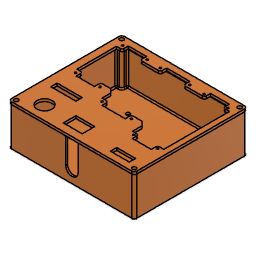
PCB Box v1 (Autodesk Fusion 360 design; units mm, degrees)
Autodesk Fusion 360 part; units mm, degrees
sketch "Sketch1" plane through (0, 0, 0) normal (0, 1, 0) x (1, 0, 0) in component "PCB_Faceplate"
  line L0 (-50, 45) -> (50, 45)
  line L1 (50, 45) -> (50, -45)
  line L2 (50, -45) -> (-50, -45)
  line L3 (-50, -45) -> (-50, 45)
  line L4 (-42.25, 38) -> (-22.75, 38) construction
  line L5 (-22.75, 38) -> (-22.75, 0.5) construction
  line L6 (-22.75, 0.5) -> (-42.25, 0.5) construction
  line L7 (-42.25, 0.5) -> (-42.25, 38) construction
  line L8 (-11.75, 37.5) -> (11.75, 37.5) construction
  line L9 (11.75, 37.5) -> (11.75, -9) construction
  line L10 (11.75, -9) -> (-11.75, -9) construction
  line L11 (-11.75, -9) -> (-11.75, 37.5) construction
  line L12 (23.75, 36.875) -> (42.75, 36.875) construction
  line L13 (42.75, 36.875) -> (42.75, -19.125) construction
  line L14 (42.75, -19.125) -> (23.75, -19.125) construction
  line L15 (23.75, -19.125) -> (23.75, 36.875) construction
  line L16 (-50, -45) -> (50, 45) construction
  circle A0 centre (-42.25, 38) radius 0.8
  circle A1 centre (-22.75, 38) radius 0.8
  circle A2 centre (-42.25, 0.5) radius 0.8
  circle A3 centre (-22.75, 0.5) radius 0.8
  circle A4 centre (-11.75, -9) radius 0.8
  circle A5 centre (11.75, -9) radius 0.8
  circle A6 centre (11.75, 37.5) radius 0.8
  circle A7 centre (-11.75, 37.5) radius 0.8
  circle A8 centre (23.75, 36.875) radius 0.8
  circle A9 centre (42.75, 36.875) radius 0.8
  circle A10 centre (42.75, -19.125) radius 0.8
  circle A11 centre (23.75, -19.125) radius 0.8
  line L17 (-44.25, 40) -> (-20.75, 40)
  line L18 (-20.75, 40) -> (-20.75, -1.5)
  line L19 (-20.75, -1.5) -> (-44.25, -1.5)
  line L20 (-44.25, -1.5) -> (-44.25, 40)
  line L21 (-14.25, 40) -> (14.25, 40)
  line L22 (14.25, 40) -> (14.25, -11.5)
  line L23 (14.25, -11.5) -> (-14.25, -11.5)
  line L24 (-14.25, -11.5) -> (-14.25, 40)
  line L25 (20.75, 40) -> (45.75, 40)
  line L26 (45.75, 40) -> (45.75, -22.25)
  line L27 (45.75, -22.25) -> (20.75, -22.25)
  line L28 (20.75, -22.25) -> (20.75, 40)
  line L29 (20.75, -22.25) -> (45.75, 40) construction
  line L30 (-14.25, -11.5) -> (14.25, 40) construction
  line L31 (-44.25, -1.5) -> (-20.75, 40) construction
  line L32 (-22.75, 0.5) -> (-42.25, 38) construction
  line L33 (-11.75, 37.5) -> (11.75, -9) construction
  line L34 (23.75, 36.875) -> (42.75, -19.125) construction
  line L35 (-20.75, 40) -> (-14.25, 40)
  line L36 (14.25, 40) -> (20.75, 40)
  line L37 (0, -45) -> (0, 45) construction
  line L38 (0, 14.25) -> (11.75, 14.25) construction
  line L39 (9.25, -11.5) -> (9.25, -6.5)
  line L40 (9.25, -6.5) -> (14.25, -6.5)
  line L41 (-9.25, -11.5) -> (-9.25, -6.5)
  line L42 (-9.25, -6.5) -> (-14.25, -6.5)
  line L43 (-25.25, -1.5) -> (-25.25, 3.5)
  line L44 (-25.25, 3.5) -> (-20.75, 3.5)
  line L45 (-39.75, -1.5) -> (-39.75, 3.5)
  line L46 (-39.75, 3.5) -> (-44.25, 3.5)
  line L47 (-44.25, 35) -> (-39.75, 35)
  line L48 (-39.75, 35) -> (-39.75, 40)
  line L49 (-25.25, 40) -> (-25.25, 35)
  line L50 (-25.25, 35) -> (-20.75, 35)
  line L51 (-14.25, 35) -> (-9.25, 35)
  line L52 (-9.25, 35) -> (-9.25, 40)
  line L53 (9.25, 40) -> (9.25, 35)
  line L54 (9.25, 35) -> (14.25, 35)
  line L55 (20.75, 35) -> (25.75, 35)
  line L56 (25.75, 35) -> (25.75, 40)
  line L57 (40.75, 40) -> (40.75, 35)
  line L58 (40.75, 35) -> (45.75, 35)
  line L59 (40.75, -22.25) -> (40.75, -17.25)
  line L60 (40.75, -17.25) -> (45.75, -17.25)
  line L61 (20.75, -17.25) -> (25.75, -17.25)
  line L62 (25.75, -17.25) -> (25.75, -22.25)
  line L63 (-20.75, 3.5) -> (-14.25, 3.5)
  line L64 (14.25, -6.5) -> (20.75, -6.5)
  line L65 (-14.25, 35) -> (-20.75, 35)
  line L66 (20.75, 35) -> (14.25, 35)
  line L67 (-42.5, -14) -> (-22.5, -14)
  line L68 (-22.5, -14) -> (-22.5, -19)
  line L69 (-22.5, -19) -> (-42.5, -19)
  line L70 (-42.5, -19) -> (-42.5, -14)
  line L71 (-42.5, -16.5) -> (-22.5, -16.5) construction
  line L72 (-32.5, -14) -> (-32.5, -1.5) construction
  line L73 (25.75, -34.75) -> (40.75, -34.75)
  line L74 (40.75, -34.75) -> (40.75, -39.75)
  line L75 (40.75, -39.75) -> (25.75, -39.75)
  line L76 (25.75, -39.75) -> (25.75, -34.75)
  line L77 (33.25, -34.75) -> (33.25, -22.25) construction
  line L78 (25.75, -37.25) -> (40.75, -37.25) construction
  circle A12 centre (-32.5, -34) radius 6
  line L79 (-12.5, -29) -> (2.5, -29)
  line L80 (2.5, -29) -> (2.5, -39)
  line L81 (2.5, -39) -> (-12.5, -39)
  line L82 (-12.5, -39) -> (-12.5, -29)
  line L83 (-47, -42) -> (-47, 42) construction
  line L84 (-47, 42) -> (47, 42) construction
  line L85 (47, 42) -> (47, -42) construction
  line L86 (47, -42) -> (-47, -42) construction
  circle A13 centre (-47, -42) radius 1.6
  circle A14 centre (47, -42) radius 1.6
  circle A15 centre (47, 42) radius 1.6
  circle A16 centre (-47, 42) radius 1.6
  line L87 (-32.5, -34) -> (-32.5, -19) construction
  line L88 (-32.5, -34) -> (-12.5, -34) construction
  dimension "d1" = 1.6
  dimension "d2" = 1.6
  dimension "d3" = 1.6
  dimension "d4" = 1.6
  dimension "d5" = 1.6
  dimension "d6" = 1.6
  dimension "d7" = 1.6
  dimension "d8" = 1.6
  dimension "d9" = 1.6
  dimension "d10" = 1.6
  dimension "d11" = 1.6
  dimension "d12" = 1.6
  dimension "d13" = 19.5
  dimension "d14" = 23.5
  dimension "d15" = 19
  dimension "d16" = 37.5
  dimension "d17" = 46.5
  dimension "d18" = 56
  dimension "d19" = 100
  dimension "d20" = 90
  dimension "d21" = 23.5
  dimension "d22" = 41.5
  dimension "d23" = 28.5
  dimension "d24" = 51.5
  dimension "d25" = 25
  dimension "d26" = 62.25
  dimension "d29" = 90
  dimension "d30" = 5
  dimension "d31" = 22.75
  dimension "d32" = 5
  dimension "d33" = 5
  dimension "d34" = 5
  dimension "d35" = 5
  dimension "d36" = 4.5
  dimension "d37" = 5
  dimension "d38" = 15
  dimension "d39" = 5
  dimension "d40" = 20
  dimension "d41" = 15
  dimension "d42" = 5
  dimension "d43" = 15
  dimension "d44" = 15
  dimension "d45" = 10
  dimension "d46" = 12
  dimension "d47" = 3
  dimension "d48" = 3.2
  dimension "d49" = 3.2
  dimension "d50" = 3.2
  dimension "d51" = 3.2
  dimension "d70" = 15
  dimension "d72" = 20
  constraint horizontal L0
  constraint vertical L1
  constraint horizontal L2
  constraint vertical L3
  constraint horizontal L4
  constraint vertical L5
  constraint horizontal L6
  constraint vertical L7
  constraint horizontal L8
  constraint vertical L9
  constraint horizontal L10
  constraint vertical L11
  constraint horizontal L12
  constraint vertical L13
  constraint horizontal L14
  constraint vertical L15
  constraint midpoint origin L16
  constraint coincident L4.start L7.end
  constraint coincident L4.end L5.start
  constraint coincident L6.end L7.start
  constraint coincident L5.end L6.start
  constraint coincident L10.end L11.start
  constraint coincident L9.end L10.start
  constraint coincident L8.end L9.start
  constraint coincident L8.start L11.end
  constraint coincident L12.start L15.end
  constraint coincident L12.end L13.start
  constraint coincident L13.end L14.start
  constraint coincident L14.end L15.start
  constraint horizontal L17
  constraint vertical L18
  constraint horizontal L19
  constraint vertical L20
  constraint horizontal L21
  constraint vertical L22
  constraint horizontal L23
  constraint vertical L24
  constraint horizontal L25
  constraint vertical L26
  constraint horizontal L27
  constraint vertical L28
  constraint midpoint L31 L32
  constraint midpoint L30 L33
  constraint midpoint L29 L34
  constraint horizontal L36
  constraint horizontal L35
  constraint equal L35 L36
  constraint midpoint L2 L37.start
  constraint midpoint L0 L37.end
  constraint midpoint L33 L38.start
  constraint midpoint L9 L38.end
  constraint coincident L37 L38.start
  constraint coincident L23 L39.start
  constraint perpendicular L23 L39
  constraint coincident L22 L40.end
  constraint perpendicular L22 L40
  constraint coincident L23 L41.start
  constraint perpendicular L23 L41
  constraint perpendicular L24 L42
  constraint coincident L24 L42.end
  constraint coincident L19 L43.start
  constraint perpendicular L19 L43
  constraint coincident L18 L44.end
  constraint perpendicular L18 L44
  constraint coincident L19 L45.start
  constraint perpendicular L19 L45
  constraint coincident L20 L46.end
  constraint perpendicular L20 L46
  constraint coincident L20 L47.start
  constraint perpendicular L20 L47
  constraint coincident L17 L48.end
  constraint perpendicular L17 L48
  constraint coincident L17 L49.start
  constraint perpendicular L17 L49
  constraint coincident L18 L50.end
  constraint perpendicular L18 L50
  constraint coincident L24 L51.start
  constraint perpendicular L24 L51
  constraint coincident L21 L52.end
  constraint perpendicular L21 L52
  constraint coincident L21 L53.start
  constraint perpendicular L21 L53
  constraint coincident L22 L54.end
  constraint perpendicular L22 L54
  constraint coincident L28 L55.start
  constraint perpendicular L15 L55
  constraint coincident L25 L56.end
  constraint perpendicular L25 L56
  constraint coincident L25 L57.start
  constraint perpendicular L12 L57
  constraint coincident L26 L58.end
  constraint perpendicular L26 L58
  constraint perpendicular L58 L59
  constraint coincident L26 L60.end
  constraint perpendicular L26 L60
  constraint coincident L27 L59.start
  constraint coincident L28 L61.start
  constraint perpendicular L15 L61
  constraint coincident L27 L62.end
  constraint perpendicular L27 L62
  constraint equal L59 L62
  constraint equal L57 L59
  constraint equal L56 L57
  constraint equal L55 L58
  constraint equal L58 L60
  constraint equal L60 L61
  constraint equal L39 L41
  constraint equal L39 L53
  constraint equal L52 L53
  constraint equal L51 L54
  constraint equal L40 L54
  constraint equal L40 L42
  constraint equal L44 L46
  constraint equal L46 L47
  constraint equal L47 L50
  constraint equal L48 L49
  constraint equal L45 L48
  constraint equal L43 L45
  constraint coincident L24 L63.end
  constraint perpendicular L24 L63
  constraint coincident L28 L64.end
  constraint perpendicular L28 L64
  constraint horizontal L65
  constraint horizontal L66
  constraint horizontal L67
  constraint vertical L68
  constraint horizontal L69
  constraint vertical L70
  constraint midpoint L70 L71.start
  constraint midpoint L68 L71.end
  constraint midpoint L67 L72.start
  constraint midpoint L19 L72.end
  constraint vertical L72
  constraint horizontal L73
  constraint vertical L74
  constraint horizontal L75
  constraint vertical L76
  constraint midpoint L73 L77.start
  constraint midpoint L27 L77.end
  constraint vertical L77
  constraint midpoint L76 L78.start
  constraint midpoint L74 L78.end
  constraint horizontal L79
  constraint vertical L80
  constraint horizontal L81
  constraint vertical L82
  constraint coincident L83.start L86.end
  constraint coincident L85.end L86.start
  constraint coincident L84.end L85.start
  constraint coincident L83.end L84.start
  constraint coincident A12.centre L87.start
  constraint midpoint L69 L87.end
  constraint vertical L87
  constraint midpoint L82 L88.end
  constraint horizontal L88
  measures "d1" diameter of A0
  measures "d2" diameter of A1
  measures "d3" diameter of A7
  measures "d4" diameter of A2
  measures "d5" diameter of A3
  measures "d6" diameter of A4
  measures "d7" diameter of A5
  measures "d8" diameter of A11
  measures "d9" diameter of A6
  measures "d10" diameter of A8
  measures "d11" diameter of A10
  measures "d12" diameter of A9
  measures "d13" distance of L4.start L4.end
  measures "d14" distance of L8.start L8.end
  measures "d15" distance of L12.start L12.end
  measures "d16" distance of L4.start L6.end
  measures "d17" distance of L8.start L10.end
  measures "d18" distance of L12.start L14.end
  measures "d19" distance of L0.start L0.end
  measures "d20" distance of L0.start L2.end
  measures "d21" distance of L17.start L17.end
  measures "d22" distance of L17.start L19.end
  measures "d23" distance of L21.start L21.end
  measures "d24" distance of L21.start L23.end
  measures "d25" distance of L25.start L25.end
  measures "d26" distance of L25.start L27.end
  measures "d29" distance of L20 L26
  measures "d30" distance of L0 L25
  measures "d31" distance of L2 L27
  measures "d32" distance of L26 L59
  measures "d33" distance of L27 L60
  measures "d34" distance of L22 L39
  measures "d35" distance of L23 L40
  measures "d36" distance of L18 L43
  measures "d37" distance of L19 L44
  measures "d38" distance of L19 L71
  measures "d39" distance of L67.end L68.end
  measures "d40" distance of L68.end L69.end
  measures "d41" distance of L74.end L75.end
  measures "d42" distance of L73.end L74.end
  measures "d43" distance of L27 L78
  measures "d44" distance of L80.end L81.end
  measures "d45" distance of L79.start L81.end
  measures "d46" diameter of A12
  measures "d48" diameter of A16
  measures "d49" diameter of A15
  measures "d50" diameter of A13
  measures "d51" diameter of A14
  measures "d70" distance of A12.centre L87.end
  measures "d72" distance of A12.centre L82
extrude "Extrude1" add sketch "Sketch1" along normal blind 2 contours L0 L1 L2 L3 | L17 L20 L47 L48 | L17 L18 L49 L50 | L19 L20 L45 L46 | L18 L24 L35 L65 | L21 L24 L51 L52 | L18 L19 L43 L44 | L21 L22 L53 L54 | L23 L24 L41 L42 | L22 L28 L36 L66 | L25 L28 L55 L56 | L22 L23 L39 L40 | L25 L26 L57 L58 | L27 L28 L61 L62 | L26 L27 L59 L60 makes body 1 in component "PCB_Faceplate"
fillet "Fillet1" radius 2 4 edges at (-50, 1, 45) (50, 1, 45) (50, 1, -45) (-50, 1, -45) on bodies 1 in component "PCB_Faceplate"
sketch "Sketch1 (2)" plane through (0, 0, 0) normal (0, 1, 0) x (1, 0, 0) in component "PCB_Box"
  line L0 (50, 43) -> (50, -43)
  arc A0 (48, -45) -> (50, -43) centre (48, -43) ccw
  line L1 (48, -45) -> (-48, -45)
  arc A1 (-50, -43) -> (-48, -45) centre (-48, -43) ccw
  line L2 (-50, -43) -> (-50, 43)
  arc A2 (-48, 45) -> (-50, 43) centre (-48, 43) ccw
  line L3 (-48, 45) -> (48, 45)
  arc A3 (50, 43) -> (48, 45) centre (48, 43) ccw
  circle A4 centre (47, 42) radius 1.6 construction
  circle A5 centre (47, -42) radius 1.6 construction
  circle A6 centre (-47, -42) radius 1.6 construction
  circle A7 centre (-47, 42) radius 1.6 construction
  line L4 (-48.5, -43) -> (-48.5, 43)
  arc A8 (-48, 43.5) -> (-48.5, 43) centre (-48, 43) ccw
  line L5 (-48, 43.5) -> (48, 43.5)
  arc A9 (48.5, 43) -> (48, 43.5) centre (48, 43) ccw
  line L6 (48.5, 43) -> (48.5, -43)
  arc A10 (48, -43.5) -> (48.5, -43) centre (48, -43) ccw
  line L7 (48, -43.5) -> (-48, -43.5)
  arc A11 (-48.5, -43) -> (-48, -43.5) centre (-48, -43) ccw
  line L8 (-50, 39) -> (-44, 39)
  line L9 (-44, 39) -> (-44, 45)
  line L10 (44, 45) -> (44, 39)
  line L11 (44, 39) -> (50, 39)
  line L12 (44, -45) -> (44, -39)
  line L13 (44, -39) -> (50, -39)
  line L14 (-50, -39) -> (-44, -39)
  line L15 (-44, -39) -> (-44, -45)
  circle A12 centre (47, -42) radius 1.1
  circle A13 centre (47, 42) radius 1.1
  circle A14 centre (-47, 42) radius 1.1
  circle A15 centre (-47, -42) radius 1.1
  dimension "d54" = 1.5
  dimension "d55" = 6
  dimension "d56" = 2.2
  dimension "d57" = 2.2
  dimension "d58" = 2.2
  dimension "d59" = 2.2
  constraint coincident L2 L8.start
  constraint perpendicular L4 L8
  constraint coincident L3 L9.end
  constraint perpendicular L3 L9
  constraint coincident L3 L10.start
  constraint perpendicular L5 L10
  constraint coincident L0 L11.end
  constraint perpendicular L0 L11
  constraint coincident L1 L12.start
  constraint perpendicular L7 L12
  constraint coincident L0 L13.end
  constraint perpendicular L0 L13
  constraint coincident L2 L14.start
  constraint perpendicular L2 L14
  constraint coincident L1 L15.end
  constraint perpendicular L1 L15
  constraint equal L14 L15
  constraint equal L12 L14
  constraint equal L12 L13
  constraint equal L8 L13
  constraint equal L8 L9
  constraint equal L9 L10
  constraint equal L10 L11
  constraint concentric A5 A12
  constraint concentric A4 A13
  constraint concentric A7 A14
  constraint concentric A6 A15
  measures "d55" distance of L12.start L12.end
  measures "d56" diameter of A14
  measures "d57" diameter of A13
  measures "d58" diameter of A15
  measures "d59" diameter of A12
extrude "Extrude1'" add sketch "Sketch1 (2)" against normal blind 30 separate body contours L0 L3 A3 L5 A9 L6 L10 L11 | L0 L6 L11 L13 | L0 A0 L1 L6 A10 L7 L12 L13 | L5 A9 L6 L10 L11 | L3 L5 L9 L10 | L6 A10 L7 L12 L13 | L2 A2 L3 L4 A8 L5 L8 L9 | L4 A8 L5 L8 L9 | L1 L7 L12 L15 | L1 A1 L2 L4 L7 A11 L14 L15 | L4 L7 A11 L14 L15 | L2 L4 L8 L14 makes body 2 in component "PCB_Box"
sketch "Sketch2" plane through (0, -30, 0) normal (0, -1, 0) x (1, 0, 0) in component "PCB_Box"
  circle A0 centre (47, -42) radius 1.1
  line L0 (-48.5, 39) -> (-44, 39)
  line L1 (-44, 39) -> (-44, 43.5)
  line L2 (-44, 43.5) -> (44, 43.5)
  line L3 (44, 43.5) -> (44, 39)
  line L4 (44, 39) -> (48.5, 39)
  line L5 (48.5, 39) -> (48.5, -39)
  line L6 (48.5, -39) -> (44, -39)
  line L7 (44, -39) -> (44, -43.5)
  line L8 (44, -43.5) -> (-44, -43.5)
  line L9 (-44, -43.5) -> (-44, -39)
  line L10 (-44, -39) -> (-48.5, -39)
  line L11 (-48.5, -39) -> (-48.5, 39)
  circle A1 centre (-47, 42) radius 1.1
  circle A2 centre (-47, -42) radius 1.1
  circle A3 centre (47, 42) radius 1.1
  arc A4 (50, 43) -> (48, 45) centre (48, 43) ccw
  line L12 (48, 45) -> (-48, 45)
  arc A5 (-48, 45) -> (-50, 43) centre (-48, 43) ccw
  line L13 (-50, 43) -> (-50, -43)
  arc A6 (-50, -43) -> (-48, -45) centre (-48, -43) ccw
  line L14 (-48, -45) -> (48, -45)
  arc A7 (48, -45) -> (50, -43) centre (48, -43) ccw
  line L15 (50, -43) -> (50, 43)
extrude "Extrude2" add sketch "Sketch2" along normal blind 1.5 contours A0 | L0 L1 L2 L3 L4 L5 L6 L7 L8 L9 L10 L11 | A1 | A2 | A3 | A4 L12 A5 L13 A6 L14 A7 L15 bodies 2 in component "PCB_Box"
fillet "Fillet1'" radius 1 8 edges at (-50, -31.5, 0) (-49.4142, -31.5, -44.4142) (0, -31.5, -45) (49.4142, -31.5, -44.4142) (50, -31.5, 0) (49.4142, -31.5, 44.4142) (0, -31.5, 45) (-49.4142, -31.5, 44.4142) on bodies 2 in component "PCB_Box"
sketch "Sketch3" plane through (0.3389, -0.4841, 45) normal (0, 0, 1) x (1, 0, 0) in component "PCB_Box"
  line L0 (-48.3389, -30.0159) -> (47.6611, -30.0159)
  line L1 (47.6611, -30.0159) -> (47.6611, 0.4841)
  line L2 (47.6611, 0.4841) -> (-48.3389, 0.4841)
  line L3 (-48.3389, 0.4841) -> (-48.3389, -30.0159)
  circle A0 centre (0, -20) radius 5
  line L4 (0, -20) -> (0, 0) construction
  line L5 (-5, -20) -> (-5, 0.4841)
  line L6 (5, -20) -> (5, 0.4841)
  dimension "d68" = 20
  dimension "d69" = 10
  constraint coincident A0.centre L4.start
  constraint coincident L4.end origin
  constraint vertical L4
  constraint coincident A0 L5.start
  constraint coincident L2 L5.end
  constraint perpendicular L2 L5
  constraint coincident A0 L6.start
  constraint coincident L2 L6.end
  constraint perpendicular L2 L6
  constraint tangent A0 L6
  constraint tangent A0 L5
  measures "d68" vertical distance of L4.end A0.centre
  measures "d69" diameter of A0
extrude "Extrude3" cut sketch "Sketch3" against normal up to surface (1.5 mm away) contours L2 A0 L5 L6 | A0 bodies 2 in component "PCB_Box"
fillet "Fillet2" radius 1.5 12 edges at (-39.75, 1, -35) (-25.25, 1, -35) (-9.25, 1, -35) (25.75, 1, -35) (9.25, 1, -35) (40.75, 1, -35) (40.75, 1, 17.25) (25.75, 1, 17.25) (9.25, 1, 6.5) (-9.25, 1, 6.5) (-25.25, 1, -3.5) (-39.75, 1, -3.5) on bodies 1 in component "PCB_Faceplate"
chamfer "Chamfer1" distance 3 angle 45 2 edges at (20.75, 1, 6.5) (-14.25, 1, -3.5) on bodies 1 in component "PCB_Faceplate"
fillet "Fillet2'" radius 2 4 edges at (-44, -15, -39) (44, -15, -39) (-44, -15, 39) (44, -15, 39) on bodies 2 in component "PCB_Box"
fillet "Fillet3" radius 1 8 edges at (44, -15, 43.5) (48.5, -15, 39) (48.5, -15, -39) (44, -15, -43.5) (-48.5, -15, -39) (-44, -15, -43.5) (-44, -15, 43.5) (-48.5, -15, 39) on bodies 2 in component "PCB_Box"
fillet "Fillet4" radius 1 2 edges at (-4.6611, 0, 44.25) (5.3389, 0, 44.25) on bodies 2 in component "PCB_Box"
fillet "Fillet5" radius 1 24 edges at (46.75, -30, -39) (44.5858, -30, -39.5858) (44, -30, -41.75) (43.7071, -30, -43.2071) (0, -30, -43.5) (-43.7071, -30, -43.2071) (-44, -30, -41.75) (-44.5858, -30, -39.5858) (-46.75, -30, -39) (-48.2071, -30, -38.7071) (-48.5, -30, 0) (-48.2071, -30, 38.7071) (-46.75, -30, 39) (-44.5858, -30, 39.5858) (-44, -30, 41.75) (-43.7071, -30, 43.2071) (0, -30, 43.5) (43.7071, -30, 43.2071) (44, -30, 41.75) (44.5858, -30, 39.5858) (46.75, -30, 39) (48.2071, -30, 38.7071) (48.5, -30, 0) (48.2071, -30, -38.7071) on bodies 2 in component "PCB_Box"
sketch "Sketch4" plane through (0, -30, 0) normal (0, 1, 0) x (-1, 0, 0) in component "PCB_Box"
  line L0 (-47.5, -38) -> (-46, -38)
  arc A0 (-43, -41) -> (-46, -38) centre (-46, -41) ccw
  line L1 (-43, -41) -> (-43, -42.5)
  line L2 (-43, -42.5) -> (43, -42.5)
  line L3 (43, -42.5) -> (43, -41)
  arc A1 (46, -38) -> (43, -41) centre (46, -41) ccw
  line L4 (46, -38) -> (47.5, -38)
  line L5 (47.5, -38) -> (47.5, 38)
  line L6 (47.5, 38) -> (46, 38)
  arc A2 (43, 41) -> (46, 38) centre (46, 41) ccw
  line L7 (43, 41) -> (43, 42.5)
  line L8 (43, 42.5) -> (-43, 42.5)
  line L9 (-43, 42.5) -> (-43, 41)
  arc A3 (-46, 38) -> (-43, 41) centre (-46, 41) ccw
  line L10 (-46, 38) -> (-47.5, 38)
  line L11 (-47.5, 38) -> (-47.5, -38)
  line L12 (25, -25) -> (-25, -25) construction
  line L13 (-25, -25) -> (-25, 25) construction
  line L14 (-25, 25) -> (25, 25) construction
  line L15 (25, 25) -> (25, -25) construction
  line L16 (25, 25) -> (-25, -25) construction
  circle A4 centre (25, -25) radius 1.5
  circle A5 centre (-25, -25) radius 1.5
  circle A6 centre (-25, 25) radius 1.5
  circle A7 centre (25, 25) radius 1.5
  dimension "d84" = 50
  dimension "d85" = 50
  dimension "d86" = 3
  dimension "d87" = 3
  dimension "d88" = 3
  dimension "d89" = 3
  constraint horizontal L12
  constraint vertical L13
  constraint horizontal L14
  constraint vertical L15
  constraint midpoint origin L16
  constraint coincident L12.start L15.end
  constraint coincident L12.end L13.start
  constraint coincident L13.end L14.start
  constraint coincident L14.end L15.start
  measures "d84" distance of L12.start L12.end
  measures "d85" distance of L12.start L14.end
  measures "d86" diameter of A4
  measures "d87" diameter of A5
  measures "d88" diameter of A7
  measures "d89" diameter of A6
extrude "Extrude4" cut sketch "Sketch4" against normal up to surface (1.5 mm away) contours A4 | A5 | A6 | A7 bodies 2 in component "PCB_Box"
sketch "Sketch2 (2)" plane through (0, 0, 0) normal (0, -1, 0) x (1, 0, 0) in component "PCB_Faceplate"
  line L0 (-17.25, -3.5) -> (-14.25, -0.5)
  line L1 (-14.25, -0.5) -> (-14.25, 6.5)
  line L2 (-14.25, 6.5) -> (-10.75, 6.5)
  arc A0 (-10.75, 6.5) -> (-9.25, 8) centre (-10.75, 8) ccw
  line L3 (-9.25, 8) -> (-9.25, 11.5)
  line L4 (-9.25, 11.5) -> (9.25, 11.5)
  line L5 (9.25, 11.5) -> (9.25, 8)
  arc A1 (9.25, 8) -> (10.75, 6.5) centre (10.75, 8) ccw
  line L6 (10.75, 6.5) -> (17.75, 6.5)
  line L7 (17.75, 6.5) -> (20.75, 9.5)
  line L8 (20.75, 9.5) -> (20.75, 17.25)
  line L9 (20.75, 17.25) -> (24.25, 17.25)
  arc A2 (24.25, 17.25) -> (25.75, 18.75) centre (24.25, 18.75) ccw
  line L10 (25.75, 18.75) -> (25.75, 22.25)
  line L11 (25.75, 22.25) -> (40.75, 22.25)
  line L12 (40.75, 22.25) -> (40.75, 18.75)
  arc A3 (40.75, 18.75) -> (42.25, 17.25) centre (42.25, 18.75) ccw
  line L13 (42.25, 17.25) -> (45.75, 17.25)
  line L14 (45.75, 17.25) -> (45.75, -35)
  line L15 (45.75, -35) -> (42.25, -35)
  arc A4 (42.25, -35) -> (40.75, -36.5) centre (42.25, -36.5) ccw
  line L16 (40.75, -36.5) -> (40.75, -40)
  line L17 (40.75, -40) -> (25.75, -40)
  line L18 (25.75, -40) -> (25.75, -36.5)
  arc A5 (25.75, -36.5) -> (24.25, -35) centre (24.25, -36.5) ccw
  line L19 (24.25, -35) -> (10.75, -35)
  arc A6 (10.75, -35) -> (9.25, -36.5) centre (10.75, -36.5) ccw
  line L20 (9.25, -36.5) -> (9.25, -40)
  line L21 (9.25, -40) -> (-9.25, -40)
  line L22 (-9.25, -40) -> (-9.25, -36.5)
  arc A7 (-9.25, -36.5) -> (-10.75, -35) centre (-10.75, -36.5) ccw
  line L23 (-10.75, -35) -> (-23.75, -35)
  arc A8 (-23.75, -35) -> (-25.25, -36.5) centre (-23.75, -36.5) ccw
  line L24 (-25.25, -36.5) -> (-25.25, -40)
  line L25 (-25.25, -40) -> (-39.75, -40)
  line L26 (-39.75, -40) -> (-39.75, -36.5)
  arc A9 (-39.75, -36.5) -> (-41.25, -35) centre (-41.25, -36.5) ccw
  line L27 (-41.25, -35) -> (-44.25, -35)
  line L28 (-44.25, -35) -> (-44.25, -3.5)
  line L29 (-44.25, -3.5) -> (-41.25, -3.5)
  arc A10 (-41.25, -3.5) -> (-39.75, -2) centre (-41.25, -2) ccw
  line L30 (-39.75, -2) -> (-39.75, 1.5)
  line L31 (-39.75, 1.5) -> (-25.25, 1.5)
  line L32 (-25.25, 1.5) -> (-25.25, -2)
  arc A11 (-25.25, -2) -> (-23.75, -3.5) centre (-23.75, -2) ccw
  line L33 (-23.75, -3.5) -> (-17.25, -3.5)
  arc A12 (-50, -43) -> (-48, -45) centre (-48, -43) ccw
  line L34 (-48, -45) -> (48, -45)
  arc A13 (48, -45) -> (50, -43) centre (48, -43) ccw
  line L35 (50, -43) -> (50, 43)
  arc A14 (50, 43) -> (48, 45) centre (48, 43) ccw
  line L36 (48, 45) -> (-48, 45)
  arc A15 (-48, 45) -> (-50, 43) centre (-48, 43) ccw
  line L37 (-50, 43) -> (-50, -43)
  line L38 (-12.5, 39) -> (2.5, 39)
  line L39 (2.5, 39) -> (2.5, 29)
  line L40 (2.5, 29) -> (-12.5, 29)
  line L41 (-12.5, 29) -> (-12.5, 39)
  circle A16 centre (11.75, -37.5) radius 0.8
  line L42 (25.75, 39.75) -> (40.75, 39.75)
  line L43 (40.75, 39.75) -> (40.75, 34.75)
  line L44 (40.75, 34.75) -> (25.75, 34.75)
  line L45 (25.75, 34.75) -> (25.75, 39.75)
  circle A17 centre (-11.75, -37.5) radius 0.8
  circle A18 centre (42.75, -36.875) radius 0.8
  circle A19 centre (11.75, 9) radius 0.8
  circle A20 centre (-42.25, -38) radius 0.8
  circle A21 centre (23.75, 19.125) radius 0.8
  circle A22 centre (23.75, -36.875) radius 0.8
  circle A23 centre (-22.75, -38) radius 0.8
  circle A24 centre (-32.5, 34) radius 6
  circle A25 centre (42.75, 19.125) radius 0.8
  circle A26 centre (-42.25, -0.5) radius 0.8
  circle A27 centre (47, 42) radius 1.6
  line L46 (-42.5, 19) -> (-22.5, 19)
  line L47 (-22.5, 19) -> (-22.5, 14)
  line L48 (-22.5, 14) -> (-42.5, 14)
  line L49 (-42.5, 14) -> (-42.5, 19)
  circle A28 centre (-47, 42) radius 1.6
  circle A29 centre (-47, -42) radius 1.6
  circle A30 centre (-22.75, -0.5) radius 0.8
  circle A31 centre (47, -42) radius 1.6
  circle A32 centre (-11.75, 9) radius 0.8
  arc A33 (-46, 39) -> (-44, 41) centre (-46, 41) ccw construction
  line L50 (-46, 39) -> (-47.5, 39) construction
  arc A34 (-47.5, 39) -> (-48.5, 38) centre (-47.5, 38) ccw construction
  line L51 (-48.5, 38) -> (-48.5, -38) construction
  line L52 (-44, 42.5) -> (-44, 41) construction
  arc A35 (-43, 43.5) -> (-44, 42.5) centre (-43, 42.5) ccw construction
  line L53 (-5.6611, 43.5) -> (-43, 43.5) construction
  line L54 (-4.6611, 43.5) -> (-5.6611, 43.5) construction
  line L55 (5.3389, 43.5) -> (-4.6611, 43.5)
  line L56 (6.3389, 43.5) -> (5.3389, 43.5) construction
  line L57 (43, 43.5) -> (6.3389, 43.5) construction
  arc A36 (44, 42.5) -> (43, 43.5) centre (43, 42.5) ccw construction
  line L58 (44, 41) -> (44, 42.5) construction
  arc A37 (44, 41) -> (46, 39) centre (46, 41) ccw construction
  line L59 (47.5, 39) -> (46, 39) construction
  arc A38 (48.5, 38) -> (47.5, 39) centre (47.5, 38) ccw construction
  line L60 (48.5, -38) -> (48.5, 38) construction
  arc A39 (47.5, -39) -> (48.5, -38) centre (47.5, -38) ccw construction
  line L61 (46, -39) -> (47.5, -39) construction
  arc A40 (46, -39) -> (44, -41) centre (46, -41) ccw construction
  line L62 (44, -42.5) -> (44, -41) construction
  arc A41 (43, -43.5) -> (44, -42.5) centre (43, -42.5) ccw construction
  line L63 (-43, -43.5) -> (43, -43.5) construction
  arc A42 (-44, -42.5) -> (-43, -43.5) centre (-43, -42.5) ccw construction
  line L64 (-44, -41) -> (-44, -42.5) construction
  arc A43 (-44, -41) -> (-46, -39) centre (-46, -41) ccw construction
  line L65 (-47.5, -39) -> (-46, -39) construction
  arc A44 (-48.5, -38) -> (-47.5, -39) centre (-47.5, -38) ccw construction
  line L66 (-4.6611, 43) -> (-5.6611, 43)
  line L67 (-5.6611, 43) -> (-43, 43)
  arc A45 (-43, 43) -> (-43.5, 42.5) centre (-43, 42.5) ccw
  line L68 (-43.5, 42.5) -> (-43.5, 41)
  arc A46 (-46, 38.5) -> (-43.5, 41) centre (-46, 41) ccw
  line L69 (-46, 38.5) -> (-47.5, 38.5)
  arc A47 (-47.5, 38.5) -> (-48, 38) centre (-47.5, 38) ccw
  line L70 (-48, 38) -> (-48, -38)
  arc A48 (-48, -38) -> (-47.5, -38.5) centre (-47.5, -38) ccw
  line L71 (-47.5, -38.5) -> (-46, -38.5)
  arc A49 (-43.5, -41) -> (-46, -38.5) centre (-46, -41) ccw
  line L72 (-43.5, -41) -> (-43.5, -42.5)
  arc A50 (-43.5, -42.5) -> (-43, -43) centre (-43, -42.5) ccw
  line L73 (-43, -43) -> (43, -43)
  arc A51 (43, -43) -> (43.5, -42.5) centre (43, -42.5) ccw
  line L74 (43.5, -42.5) -> (43.5, -41)
  arc A52 (46, -38.5) -> (43.5, -41) centre (46, -41) ccw
  line L75 (46, -38.5) -> (47.5, -38.5)
  arc A53 (47.5, -38.5) -> (48, -38) centre (47.5, -38) ccw
  line L76 (48, -38) -> (48, 38)
  arc A54 (48, 38) -> (47.5, 38.5) centre (47.5, 38) ccw
  line L77 (47.5, 38.5) -> (46, 38.5)
  arc A55 (43.5, 41) -> (46, 38.5) centre (46, 41) ccw
  line L78 (43.5, 41) -> (43.5, 42.5)
  arc A56 (43.5, 42.5) -> (43, 43) centre (43, 42.5) ccw
  line L79 (43, 43) -> (6.3389, 43)
  line L80 (6.3389, 43) -> (5.3389, 43)
  line L81 (5.3389, 43) -> (-4.6611, 43)
  line L82 (-4.6611, 41.5) -> (-5.6611, 41.5)
  line L83 (-5.6611, 41.5) -> (-42, 41.5)
  line L84 (-42, 41.5) -> (-42, 41)
  arc A57 (-46, 37) -> (-42, 41) centre (-46, 41) ccw
  line L85 (-46, 37) -> (-46.5, 37)
  line L86 (-46.5, 37) -> (-46.5, -37)
  line L87 (-46.5, -37) -> (-46, -37)
  arc A58 (-42, -41) -> (-46, -37) centre (-46, -41) ccw
  line L88 (-42, -41) -> (-42, -41.5)
  line L89 (-42, -41.5) -> (42, -41.5)
  line L90 (42, -41.5) -> (42, -41)
  arc A59 (46, -37) -> (42, -41) centre (46, -41) ccw
  line L91 (46, -37) -> (46.5, -37)
  line L92 (46.5, -37) -> (46.5, 37)
  line L93 (46.5, 37) -> (46, 37)
  arc A60 (42, 41) -> (46, 37) centre (46, 41) ccw
  line L94 (42, 41) -> (42, 41.5)
  line L95 (42, 41.5) -> (6.3389, 41.5)
  line L96 (6.3389, 41.5) -> (5.3389, 41.5)
  line L97 (5.3389, 41.5) -> (-4.6611, 41.5)
  dimension "d92" = -0.5
  dimension "d93" = -2
extrude "Extrude2'" add sketch "Sketch2 (2)" along normal blind 2 contours L66 L67 A45 L68 A46 L69 A47 L70 A48 L71 A49 L72 A50 L73 A51 L74 A52 L75 A53 L76 A54 L77 A55 L78 A56 L79 L80 L81 bodies 1 in component "PCB_Faceplate"
chamfer "Chamfer2" distance 0.5 angle 45 24 edges at (0, -2, 43) (-43.3536, -2, 42.8536) (-43.5, -2, 41.75) (-44.2322, -2, 39.2322) (-46.75, -2, 38.5) (-47.8536, -2, 38.3536) (-48, -2, 0) (-47.8536, -2, -38.3536) (-46.75, -2, -38.5) (-44.2322, -2, -39.2322) (-43.5, -2, -41.75) (-43.3536, -2, -42.8536) (0, -2, -43) (43.3536, -2, -42.8536) (43.5, -2, -41.75) (44.2322, -2, -39.2322) (46.75, -2, -38.5) (47.8536, -2, -38.3536) (48, -2, 0) (47.8536, -2, 38.3536) (46.75, -2, 38.5) (44.2322, -2, 39.2322) (43.5, -2, 41.75) (43.3536, -2, 42.8536) on bodies 1 in component "PCB_Faceplate"
component "PCB_Faceplate" placed x (1, 0, 0) y (0, 1, 0) z (0, 0, 1) at (0, 0, 0)
component "PCB_Box" placed x (1, 0, 0) y (0, 1, 0) z (0, 0, 1) at (0, 0, 0)
equation "d2 = d1"
equation "d3 = d1"
equation "d4 = d1"
equation "d5 = d1"
equation "d6 = d1"
equation "d7 = d1"
equation "d8 = d1"
equation "d9 = d1"
equation "d10 = d1"
equation "d11 = d1"
equation "d12 = d1"
equation "d49 = d48"
equation "d50 = d48"
equation "d51 = d48"
equation "d57 = d56"
equation "d58 = d56"
equation "d59 = d56"
equation "d87 = d86"
equation "d88 = d86"
equation "d89 = d86"
